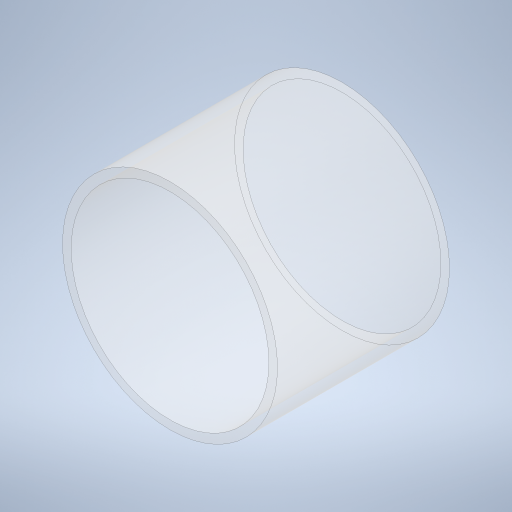
# Autodesk Inventor part: camera_pipe
Saved by Autodesk Inventor 2024 (Build 280153000, 153)
## iProperties
Created: 2025-05-20
Part Number: camera_pipe
Material: Tworzywo sztuczne ABS
Document SubType Name: Modeling
Designer: Paweł
Density: 1.06 g/cm^3
Appearance: Gładki — biały
Mass: 13 g
Surface Area: 102.102 cm^2
Volume: 78.5398 cm^3
Author: Paweł
Autodesk Inventor part; units mm, degrees
ref_plane "YZ Plane" through (0, 0, 0) normal (1, 0, 0) x (0, 1, 0)
ref_plane "XZ Plane" through (0, 0, 0) normal (0, 1, 0) x (-1, 0, 0)
ref_plane "XY Plane" through (0, 0, 0) normal (0, 0, 1) x (1, 0, 0)
sketch "Szkic1" plane through (0, 0, 0) normal (0, 0, 1) x (1, 0, 0)
  circle A0 centre (0, 0) radius 25
  circle A1 centre (0, 0) radius 23
  dimension "d0" = 50
  dimension "d1" = 46
  constraints: 2 centre point, 2 coincident
  measures "d0" diameter of A0
  measures "d1" diameter of A1
extrude "Wyciągnięcie proste1" add sketch "Szkic1" along normal blind 40
